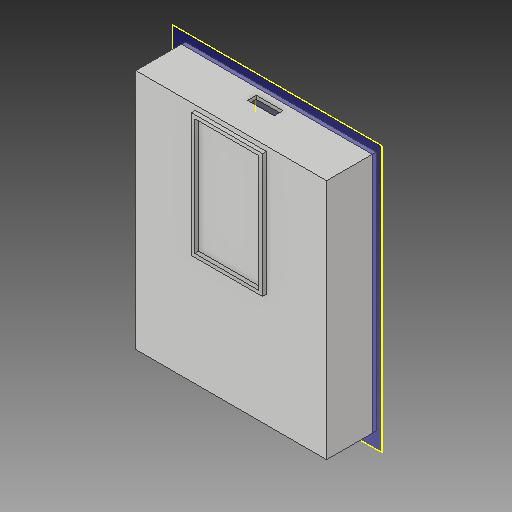
# Autodesk Inventor part: box_low
Saved by Autodesk Inventor 2019 (Build 230136000, 136)
## iProperties
Created: 2020-06-11
Part Number: box_low
Material: Generic
Document SubType Name: Modeling
Designer: assman
Density: 1 g/cm^3
Appearance: Default
Author: assman
Autodesk Inventor part; units mm, degrees
ref_plane "YZ Plane" through (0, 0, 0) normal (1, 0, 0) x (0, 1, 0)
sketch "Sketch1" plane through (0, 0, 0) normal (0, 0, 1) x (1, 0, 0)
  line L0 (-9, 16.5) -> (9, 16.5) construction
  line L1 (9, 16.5) -> (9, -16.5) construction
  line L2 (-9, -16.5) -> (-9, 16.5) construction
  line L3 (9, -16.5) -> (-9, -16.5) construction
  line L4 (9.1, 16.6) -> (-9.1, 16.6)
  line L5 (-9.1, 16.6) -> (-9.1, -16.6)
  line L6 (-9.1, -16.6) -> (9.1, -16.6)
  line L7 (9.1, -16.6) -> (9.1, 16.6)
  line L8 (10.1, 17.6) -> (-10.1, 17.6)
  line L9 (-10.1, 17.6) -> (-10.1, -17.6)
  line L10 (-10.1, -17.6) -> (10.1, -17.6)
  line L11 (10.1, -17.6) -> (10.1, 17.6)
  point P0 (0, 0)
  dimension "d0" = 0.1
  dimension "d1" = 1
  constraints: 16 end point, 6 other
  measures "d0" distance between parallel lines of L0 L4
  measures "d1" distance between parallel lines of L7 L11
extrude "Extrusion1" add sketch "Sketch1" along normal mid plane 16.35
sketch "Sketch2" plane through (-10.1, -17.6, 8.175) normal (0, -1, 0) x (1, 0, 0)
  point P0 (10.1, -8.175)
  point P1 (10.1, -8.175)
  constraints: 1 coincident
ref_plane "Work Plane1" through (-18.25, -49.8, 6.05) normal (0, 0, 1) x (1, 0, 0)
sketch "Sketch3" plane through (-18.25, -49.8, 6.05) normal (0, 0, 1) x (1, 0, 0)
  line L0 (36.5, 14) -> (0, 14) construction
  line L1 (36.5, 14) -> (36.5, 22.2) construction
  line L2 (0, 22.2) -> (36.5, 22.2) construction
  line L3 (0, 14) -> (0, 22.2) construction
  line L4 (40.5, 0) -> (-4, 0) construction
  line L5 (-4, 0) -> (-4, 14) construction
  line L6 (40.5, 14) -> (-4, 14) construction
  line L7 (40.5, 0) -> (40.5, 14) construction
  line L8 (40.5, 0) -> (-4, 0)
  line L9 (-4, 0) -> (-8.7761, 0)
  line L10 (40.5, 0) -> (45.5, 0)
  line L11 (45.5, 0) -> (45.5, 67.4)
  line L12 (-8.7761, 67.4) -> (-8.7761, 0)
  line L13 (14.45, 68.75) -> (22.05, 68.75) construction
  line L14 (-8.7761, 67.4) -> (-8.7761, 68.75)
  line L15 (-8.7761, 68.75) -> (45.5, 68.75)
  line L16 (45.5, 68.75) -> (45.5, 67.4)
  point P0 (18.25, 49.8)
  dimension "d4" = 5
  constraints: 16 end point, 2 horizontal, 2 point on line, 1 perpendicular, 1 vertical
  measures "d4" distance of L4.start L10.end
extrude "Extrusion2" add sketch "Sketch3" along normal blind 1
sketch "Sketch4" plane through (-18.25, -49.8, 6.05) normal (0, 0, -1) x (-1, 0, 0)
  line L0 (-27.35, 33.2) -> (-27.35, 66.4) projected
  line L1 (-27.35, 66.4) -> (-9.15, 66.4) projected
  line L2 (-9.15, 66.4) -> (-9.15, 33.2) projected
  line L3 (-9.15, 33.2) -> (-27.35, 33.2) projected
  line L4 (-8.15, 67.4) -> (-28.35, 67.4) projected
  line L5 (-28.35, 67.4) -> (-28.35, 32.2) projected
  line L6 (-28.35, 32.2) -> (-8.15, 32.2) projected
  line L7 (-8.15, 32.2) -> (-8.15, 67.4) projected
  point P0 (-18.25, 49.8)
extrude "Extrusion3" [suppressed]
sketch "Sketch5" plane through (-18.25, -49.8, 6.05) normal (0, 0, -1) x (-1, 0, 0)
  line L0 (8.7761, 68.75) -> (-45.5, 68.75) projected
  line L1 (-45.5, 68.75) -> (-45.5, 0) projected
  line L2 (8.7761, 0) -> (8.7761, 68.75) projected
  line L3 (-45.5, 0) -> (8.7761, 0) projected
  line L4 (-44.5, 67.75) -> (7.7761, 67.75)
  line L5 (7.7761, 67.75) -> (7.7761, 1)
  line L6 (7.7761, 1) -> (-44.5, 1)
  line L7 (-44.5, 1) -> (-44.5, 67.75)
  point P0 (-18.25, 49.8)
  dimension "d9" = 1
  constraints: 8 end point, 3 other
  measures "d9" distance between parallel lines of L0 L4
ref_plane "Work Plane2" through (-22.25, -49.8, -5.95) normal (0, 0, -1) x (0, 1, 0)
extrude "Extrusion4" add sketch "Sketch5" along normal up to surface (12 mm away)
sketch "Sketch6" plane through (-27.0261, -49.8, 7.05) normal (0, -1, 0) x (1, 0, 0)
  arc A0 (8.7761, -1.1) -> (4.7761, -5.1) centre (8.7761, -5.1) ccw projected
  line L0 (4.7761, -13) -> (4.7761, -5.1) projected
  line L1 (8.7761, -1.1) -> (45.2761, -1.1) projected
  arc A1 (49.2761, -5.1) -> (45.2761, -1.1) centre (45.2761, -5.1) ccw projected
  line L2 (49.2761, -5.1) -> (49.2761, -13) projected
  line L3 (0, -13) -> (54.2761, -13) construction
  line L4 (49.2761, -13) -> (4.7761, -13)
  line L5 (54.2761, -13) -> (0, -13) projected
  point P0 (27.0261, -7.05)
  constraints: 2 end point, 1 collinear, 1 other
extrude "Extrusion5" cut sketch "Sketch6" against normal blind 1
ref_plane "Work Plane3" through (27.25, 18.95, -6.05) normal (0, 0, -1) x (-1, 0, 0)
sketch "Sketch7" plane through (27.25, 18.95, -6.05) normal (0, 0, -1) x (-1, 0, 0)
  line L0 (54.2761, 0) -> (54.2761, -68.75) projected
  line L1 (0, 0) -> (54.2761, 0) projected
  line L2 (0, -68.75) -> (0, 0) projected
  line L3 (5, -68.75) -> (0, -68.75) projected
  line L4 (54.2761, -68.75) -> (49.5, -68.75) projected
  line L5 (5, -68.75) -> (49.5, -68.75)
  line L6 (9, -67.75) -> (45.5, -67.75) projected
  point P0 (27.25, -18.95)
  constraints: 2 end point, 1 parallel
extrude "Extrusion6" add sketch "Sketch7" along normal blind 1 and the other way blind 0.1
sketch "Sketch8" plane through (-27.0261, 18.95, 7.05) normal (0, 1, 0) x (1, 0, 0)
  line L0 (23.2261, 11.05) -> (30.8261, 11.05) projected
  line L1 (23.2261, 8.55) -> (23.2261, 11.05) projected
  line L2 (30.8261, 8.55) -> (30.8261, 11.05) projected
  line L3 (23.2261, 8.55) -> (30.8261, 8.55) projected
  point P0 (27.0261, 7.05)
extrude "Extrusion7" cut sketch "Sketch8" against normal blind 1
ref_plane "Work Plane4" through (27.25, 18.95, -5.95) normal (0, 0, -1) x (-1, 0, 0)
split body "Split1" result two bodies by plane through (27.25, 18.95, -5.95) normal (0, 0, -1) first body at (3.4413, -39.0667, -6.55)
sketch "Sketch9" plane through (0, 0, -8.175) normal (0, 0, -1) x (-1, 0, 0)
  line L0 (-9.1, -16.6) -> (-9.1, 16.6) projected
  line L1 (-9.1, 16.6) -> (9.1, 16.6) projected
  line L2 (9.1, 16.6) -> (9.1, -16.6) projected
  line L3 (9.1, -16.6) -> (-9.1, -16.6) projected
  line L4 (10.1, 17.6) -> (-10.1, 17.6) projected
  line L5 (-10.1, 17.6) -> (-10.1, -17.6) projected
  line L6 (-10.1, -17.6) -> (10.1, -17.6) projected
  line L7 (10.1, -17.6) -> (10.1, 17.6) projected
  point P0 (0, 0)
ref_plane "Work Plane5" through (-9, -16.5, -1.5) normal (0, 0, -1) x (0, 1, 0)
extrude "Extrusion8" cut sketch "Sketch9" against normal up to surface (6.675 mm away) bodies 3
body "Solid2"
body "Solid3"
